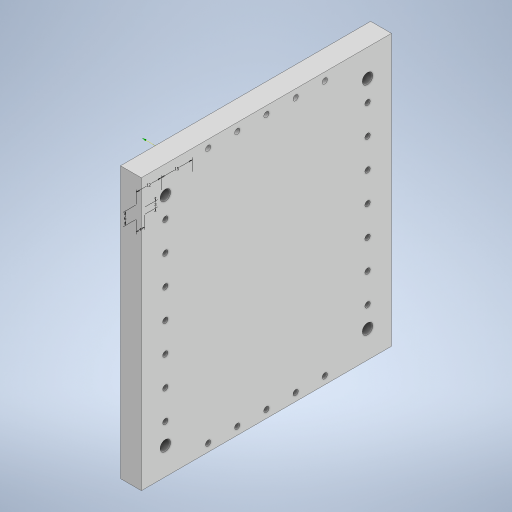
# Autodesk Inventor part: Soporte PCB
Saved by Autodesk Inventor 2023 (Build 270158000, 158)
## iProperties
Created: 2023-02-25
Part Number: Soporte PCB
Material: Genérico
Document SubType Name: Modeling
Designer: sergi
Density: 1 g/cm^3
Appearance: Valor por defecto
Author: sergi
Autodesk Inventor part; units mm, degrees
ref_plane "YZ Plane" through (0, 0, 0) normal (1, 0, 0) x (0, 1, 0)
ref_plane "XZ Plane" through (0, 0, 0) normal (0, 1, 0) x (-1, 0, 0)
ref_plane "XY Plane" through (0, 0, 0) normal (0, 0, 1) x (1, 0, 0)
sketch "Boceto1" plane through (0, 0, 0) normal (1, 0, 0) x (0, 1, 0)
  line L0 (-57.5, -42.7876) -> (57.5, -42.7876)
  line L1 (57.5, -42.7876) -> (57.5, 42.2124)
  line L2 (57.5, 42.2124) -> (-57.5, 42.2124)
  line L3 (-57.5, 42.2124) -> (-57.5, -42.7876)
  line L4 (-57.5, -42.7876) -> (57.5, 42.2124) construction
  line L5 (57.5, -42.7876) -> (-57.5, 42.2124) construction
  point P0 (0, 0)
  point P1 (0, -0.2876)
  dimension "d0" = 115
  dimension "d1" = 85
  constraints: 12 end point, 2 midpoint, 2 parallel, 1 horizontal, 1 perpendicular
  measures "d0" distance of L2.end L1.end
  measures "d1" distance of L1.end L0.end
sketch "Boceto2" plane through (0, 0, 0) normal (1, 0, 0) x (0, 1, 0)
  line L0 (-65, -60) -> (65, -60)
  line L1 (65, -60) -> (65, 60)
  line L2 (65, 60) -> (-65, 60)
  line L3 (-65, 60) -> (-65, -60)
  line L4 (-65, -60) -> (65, 60) construction
  line L5 (65, -60) -> (-65, 60) construction
  point P0 (0, 0)
  dimension "d2" = 130
  dimension "d3" = 120
  constraints: 12 end point, 2 midpoint, 2 parallel, 1 horizontal, 1 perpendicular
  measures "d2" distance of L2.end L1.end
  measures "d3" distance of L1.end L0.end
extrude "Extrusión1" add sketch "Boceto2" along normal blind 10
extrude "Extrusión2" cut sketch "Boceto1" along normal blind 2
sketch "Boceto3" plane through (0, 0, 0) normal (-1, 0, 0) x (0, 0, 1)
  line L0 (0, 0) -> (0, -52)
  line L1 (0, 0) -> (0, 52)
  line L2 (-60, -65) -> (-60, 65) projected
  line L3 (0, -52) -> (46, -52)
  line L4 (0, -52) -> (-46, -52)
  line L5 (-46, -52) -> (-48.5, -52)
  circle A0 centre (-48.5, -52) radius 2.5
  line L6 (46, -52) -> (48.5, -52)
  circle A1 centre (48.5, -52) radius 2.5
  line L7 (0, 52) -> (48.5, 52)
  line L8 (0, 52) -> (-48.5, 52)
  line L9 (-42.7876, -57.5) -> (-42.7876, 57.5) projected
  circle A2 centre (-48.5, 52) radius 2.5
  circle A3 centre (48.5, 52) radius 2.5
  dimension "d8" = 52
  dimension "d9" = 52
  dimension "d10" = 46
  dimension "d11" = 46
  dimension "d12" = 2.5
  dimension "d13" = 2.5
  dimension "d14" = 48.5
  dimension "d15" = 5
  dimension "d16" = 5
  constraints: 16 end point, 4 coincident, 3 horizontal, 2 centre point, 2 horizontal alignment, 2 perpendicular, 2 vertical, 4 other
  measures "d8" distance of L0.start L0.end
  measures "d9" distance of L0.start L1.end
  measures "d10" distance of L0.end L3.end
  measures "d11" distance of L0.end L4.end
  measures "d12" distance of L4.end L5.end
  measures "d13" distance of L3.end L6.end
  measures "d14" distance of L1.end L7.end
  measures "d15" diameter of A2
  measures "d16" diameter of A3
extrude "Extrusión3" cut sketch "Boceto3" against normal through all contours A1 | A0 | A2 | A3
chamfer "Chaflán1" distance 2.3 angle 45 4 edges at (0, 52, -51) (0, -52, -51) (0, -52, 46) (0, 52, 46)
sketch "Boceto5" plane through (0, 0, 0) normal (-1, 0, 0) x (0, 0, 1)
  circle A0 centre (-48.5, 52) radius 2.5 projected
  circle A1 centre (-48.5, -52) radius 2.5 projected
  line L0 (-48.5, 52) -> (-48.5, -52)
  line L1 (-48.5, 52) -> (-48.5, 44)
  line L2 (-48.5, 52) -> (-48.5, 38)
  circle A2 centre (-48.5, 0) radius 1.25
  circle A3 centre (-48.5, -14) radius 1.25
  circle A4 centre (-48.5, -28) radius 1.25
  circle A5 centre (-48.5, 14) radius 1.25
  circle A6 centre (-48.5, 28) radius 1.25
  circle A7 centre (-48.5, 42) radius 1.25
  line L3 (-48.5, -28) -> (-48.5, -42)
  circle A8 centre (-48.5, -42) radius 1.25
  line L4 (0, 0) -> (0, -23.0144)
  circle A9 centre (48.5, 0) radius 1.25
  circle A10 centre (48.5, -14) radius 1.25
  circle A11 centre (48.5, -28) radius 1.25
  circle A12 centre (48.5, 14) radius 1.25
  circle A13 centre (48.5, 28) radius 1.25
  circle A14 centre (48.5, 42) radius 1.25
  circle A15 centre (48.5, -42) radius 1.25
  dimension "d27" = 2.5
  dimension "d30" = 14
  dimension "d37" = 14
  dimension "d42" = 14
  dimension "d43" = 2.5
  constraints: 14 centre point, 10 end point, 7 symmetric about line, 3 point on line, 3 vertical, 1 coincident, 1 midpoint, 17 other
  measures "d27" diameter of A2
  measures "d30" distance of A2.centre A3.centre
  measures "d37" distance of A2.centre A5.centre
  measures "d42" distance of L3.start L3.end
  measures "d43" diameter of A8
extrude "Extrusión4" cut sketch "Boceto5" against normal through all contours A8 L0 | L0 A8 | A4 L0 | L0 A4 | A3 L0 | L0 A3 | A2 L0 | L0 A2 | A5 L0 | L0 A5 | A6 L0 | L0 A6 | A7 L0 | L0 A7 | A9 | A10 | A11 | A12 | A13 | A14 | A15
sketch "Boceto6" plane through (0, 0, 0) normal (-1, 0, 0) x (0, 0, 1)
  line L0 (60, -65) -> (-60, -65) projected
  line L1 (42.2124, -57.5) -> (-42.7876, -57.5) projected
  line L2 (0, -57.5) -> (0, -65)
  circle A0 centre (0, -61.25) radius 1.25
  circle A1 centre (-14, -61.25) radius 1.25
  circle A2 centre (-28, -61.25) radius 1.25
  circle A3 centre (14, -61.25) radius 1.25
  circle A4 centre (28, -61.25) radius 1.25
  line L3 (0, 0) -> (18.5256, 0)
  circle A5 centre (0, 61.25) radius 1.25
  circle A6 centre (-14, 61.25) radius 1.25
  circle A7 centre (-28, 61.25) radius 1.25
  circle A8 centre (14, 61.25) radius 1.25
  circle A9 centre (28, 61.25) radius 1.25
  dimension "d46" = 2.5
  dimension "d49" = 14
  dimension "d56" = 14
  constraints: 10 centre point, 5 symmetric about line, 4 end point, 3 horizontal, 2 midpoint, 1 point on line, 13 other
  measures "d46" diameter of A0
  measures "d49" distance of A0.centre A1.centre
  measures "d56" distance of A0.centre A3.centre
extrude "Extrusión5" cut sketch "Boceto6" against normal through all
sketch "Boceto7" plane through (0, 0, 0) normal (-1, 0, 0) x (0, 0, 1)
  circle A0 centre (48.5, 42) radius 1.25 projected
  line L0 (48.5, 42) -> (48.5, 39)
  line L1 (48.5, 39) -> (52.5, 39)
  line L2 (52.5, 39) -> (52.5, 45)
  line L3 (52.5, 45) -> (40.5, 45)
  line L4 (40.5, 45) -> (25.5, 45)
  point P0 (0, 0)
  dimension "d63" = 3
  dimension "d64" = 4
  dimension "d65" = 6
  dimension "d66" = 12
  dimension "d67" = 15
  constraints: 10 end point, 3 perpendicular, 1 point on line, 1 vertical
  measures "d63" distance of L0.start L0.end
  measures "d64" distance of L0.end L1.end
  measures "d65" distance of L1.end L2.end
  measures "d66" distance of L2.end L3.end
  measures "d67" distance of L3.end L4.end
